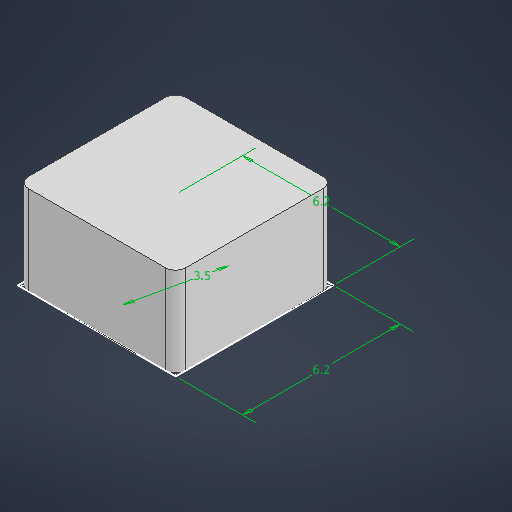
# Autodesk Inventor part: Button
Saved by Autodesk Inventor 2026.2 (Build 302298000, 298)
## iProperties
Created: 2026-03-12
Part Number: Button
Material: Generic
Document SubType Name: Modeling
Designer: Cobble
Density: 1 g/cm^3
Appearance: Default
Author: Cobble
Autodesk Inventor part; units mm, degrees
ref_plane "YZ Plane" through (0, 0, 0) normal (1, 0, 0) x (0, 1, 0)
ref_plane "XZ Plane" through (0, 0, 0) normal (0, 1, 0) x (-1, 0, 0)
ref_plane "XY Plane" through (0, 0, 0) normal (0, 0, 1) x (1, 0, 0)
sketch "Sketch1" plane through (0, 0, 0) normal (0, 0, 1) x (1, 0, 0)
  line L0 (0, 0) -> (6.2, 0)
  line L1 (6.2, 0) -> (6.2, 6.2)
  line L2 (6.2, 6.2) -> (0, 6.2)
  line L3 (0, 6.2) -> (0, 0)
  line L4 (0, 6.2) -> (6.2, 0) construction
  line L5 (6.2, 6.2) -> (0, 0) construction
  circle A0 centre (3.1, 3.1) radius 1.75
  dimension "d0" = 6.2
  dimension "d1" = 6.2
  dimension "d2" = 3.5
  constraints: 12 end point, 2 parallel, 1 centre point, 1 horizontal, 1 midpoint, 1 perpendicular
  measures "d0" distance of L2.end L1.end
  measures "d1" distance of L1.end L0.end
  measures "d2" diameter of A0
extrude "Extrusion1" add sketch "Sketch1" along normal blind 3.5 contours L3 L2 L1 L0 | A0
extrude "Extrusion2" add sketch "Sketch1" against normal blind 1.5 contours A0
fillet "Fillet1" radius 0.4 4 edges at (0, 6.2, 1.75) (0, 0, 1.75) (6.2, 0, 1.75) (6.2, 6.2, 1.75)
fillet "Fillet2" radius 0.25 1 edges at (1.35, 3.1, -1.5)
body "Solid1"
